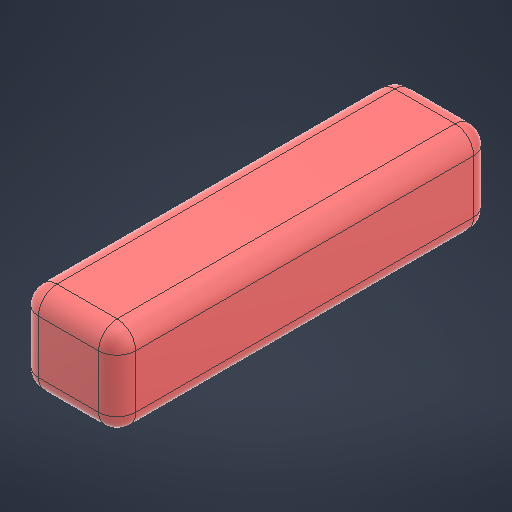
# Autodesk Inventor part: 5V_LIon
Saved by Autodesk Inventor 2026 (Build 300175050, 175E)
## iProperties
Created: 2025-06-14
Part Number: 5V_LIon
Material: Generic
Document SubType Name: Modeling
Designer: satom
Density: 1 g/cm^3
Appearance: Default
Author: satom
Autodesk Inventor part; units mm, degrees
ref_plane "YZ Plane" through (0, 0, 0) normal (1, 0, 0) x (0, 1, 0)
ref_plane "XZ Plane" through (0, 0, 0) normal (0, 1, 0) x (-1, 0, 0)
ref_plane "XY Plane" through (0, 0, 0) normal (0, 0, 1) x (1, 0, 0)
sketch "Sketch1" plane through (0, 0, 0) normal (0, 0, 1) x (1, 0, 0)
  line L0 (-13.335, 12.3825) -> (13.335, 12.3825)
  line L1 (13.335, 12.3825) -> (13.335, -12.3825)
  line L2 (13.335, -12.3825) -> (-13.335, -12.3825)
  line L3 (-13.335, -12.3825) -> (-13.335, 12.3825)
  line L4 (-13.335, 12.3825) -> (13.335, -12.3825) construction
  line L5 (13.335, 12.3825) -> (-13.335, -12.3825) construction
  point P0 (0, 0)
  dimension "d0" = 26.67
  dimension "d1" = 24.765
  constraints: 12 end point, 2 midpoint, 2 parallel, 1 horizontal, 1 perpendicular
  measures "d0" distance of L1.end L2.end
  measures "d1" distance of L0.end L1.end
extrude "Extrusion1" add sketch "Sketch1" along normal blind 102.87
fillet "Fillet1" radius 5.08 12 edges at (13.335, 12.3825, 51.435) (13.335, 0, 102.87) (0, 12.3825, 102.87) (0, -12.3825, 102.87) (13.335, -12.3825, 51.435) (-13.335, 0, 102.87) (13.335, 0, 0) (0, 12.3825, 0) (-13.335, 0, 0) (0, -12.3825, 0) (-13.335, 12.3825, 51.435) (-13.335, -12.3825, 51.435)
sketch "Sketch2" plane through (0, 0, 0) normal (0, 0, -1) x (-1, 0, 0)
  line L0 (-5.715, -0.1905) -> (5.715, -0.1905)
  line L1 (5.715, -0.1905) -> (5.715, -4.7625)
  line L2 (5.715, -4.7625) -> (-5.715, -4.7625)
  line L3 (-5.715, -4.7625) -> (-5.715, -0.1905)
  line L4 (-8.255, -12.3825) -> (8.255, -12.3825) projected
  line L5 (-8.255, 12.3825) -> (8.255, 12.3825) construction
  line L6 (0, 12.3825) -> (0, -12.3825) construction
  line L7 (-3.556, 4.8895) -> (3.556, 4.8895)
  line L8 (3.556, 4.8895) -> (3.556, 3.6195)
  line L9 (-3.556, 4.8895) -> (-3.556, 3.6195)
  line L10 (-2.54, 2.3495) -> (2.54, 2.3495)
  line L11 (2.54, 2.3495) -> (3.556, 3.6195)
  line L12 (-3.556, 3.6195) -> (-2.54, 2.3495)
  point P0 (0, 0)
  dimension "d5" = 11.43
  dimension "d6" = 4.572
  dimension "d7" = 7.62
  dimension "d8" = 5.715
  dimension "d9" = 7.112
  dimension "d10" = 1.27
  dimension "d11" = 1.27
  dimension "d12" = 5.08
  dimension "d13" = 2.54
  dimension "d14" = 1.016
  dimension "d15" = 3.556
  dimension "d16" = 2.54
  constraints: 22 end point, 3 horizontal, 2 midpoint, 2 parallel, 2 perpendicular, 1 vertical
  measures "d5" distance of L1.end L2.end
  measures "d6" distance of L2.end L0.start
  measures "d7" distance between parallel lines of L4 L2
  measures "d8" distance between parallel lines of L1 L6
  measures "d9" distance of L7.start L7.end
  measures "d10" distance of L7.end L8.end
  measures "d11" distance of L7.start L9.end
  measures "d12" distance of L10.start L10.end
  measures "d13" distance between parallel lines of L10 L7
  measures "d14" horizontal distance of L8.end L10.end
  measures "d15" distance between parallel lines of L8 L6
  measures "d16" distance between parallel lines of L0 L10
extrude "Extrusion2" cut sketch "Sketch2" against normal blind 12.7
equation "\"d8\" = 0.5 * d5"
equation "\"d15\" = 0.5 * d9"
body "Solid1"
